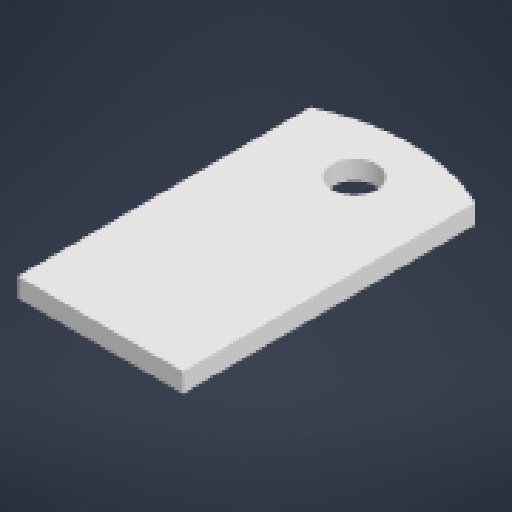
# Autodesk Inventor part: gasket_2
Saved by Autodesk Inventor 2024 (Build 280153000, 153)
## iProperties
Created: 2023-11-08
Part Number: gasket_2
Material: Типовые
Document SubType Name: Modeling
Designer: user
Density: 1 g/cm^3
Appearance: По умолчанию
Author: user
Autodesk Inventor part; units mm, degrees
ref_plane "YZ Plane" through (0, 0, 0) normal (1, 0, 0) x (0, 1, 0)
ref_plane "XZ Plane" through (0, 0, 0) normal (0, 1, 0) x (-1, 0, 0)
ref_plane "XY Plane" through (0, 0, 0) normal (0, 0, 1) x (1, 0, 0)
sketch "Эскиз1" plane through (0, 0, 0) normal (0, 0, 1) x (1, 0, 0)
  circle A0 centre (-7, 12) radius 1.5 projected
  circle A1 centre (0, 5) radius 1.5 projected
  circle A2 centre (7, 12) radius 1.5 projected
  circle A3 centre (7, 40) radius 1.5 projected
  circle A4 centre (-7, 40) radius 1.5 projected
  point P0 (0, 0)
extrude "Выдавливание1" add sketch "Эскиз1" against normal blind 3
sketch "Эскиз3" plane through (0, 5, 0) normal (0, 0, 1) x (1, 0, 0)
  line L0 (-13, -5) -> (-13, 37.6484)
  line L1 (13, 37.6484) -> (13, -5)
  line L2 (13, -5) -> (-13, -5)
  circle A0 centre (0, 35) radius 3.5
  arc A1 (13, 37.6484) -> (9.6, 42.3855) centre (8, 37.6484) ccw
  arc A2 (9.6, 42.3855) -> (-9.6, 42.3855) centre (0, 13.963) ccw
  arc A3 (-9.6, 42.3855) -> (-13, 37.6484) centre (-8, 37.6484) ccw
  point P0 (0, -5)
extrude "Выдавливание2" add sketch "Эскиз3" along normal blind 3
